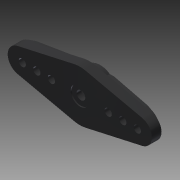
# Autodesk Inventor part: servo arm TGY-S8166M double
Saved by Autodesk Inventor 2013 (Build 170138000, 138)
## iProperties
Created: 2014-10-10
Part Number: servo arm TGY-S8166M double
Material: Acetal Resin, Black
Document SubType Name: Modeling
Designer: Masta
Density: 1.425 g/cm^3
Mass: 3.25867 g
Surface Area: 21.815 cm^2
Volume: 2.28679 cm^3
Author: Masta
Autodesk Inventor part; units mm, degrees
ref_plane "YZ Plane" through (0, 0, 0) normal (1, 0, 0) x (0, 1, 0)
ref_plane "XZ Plane" through (0, 0, 0) normal (0, 1, 0) x (-1, 0, 0)
ref_plane "XY Plane" through (0, 0, 0) normal (0, 0, 1) x (1, 0, 0)
sketch "Sketch1" plane through (0, 0, 0) normal (0, 1, 0) x (-1, 0, 0)
  line L0 (0, 0) -> (0, 8.7)
  arc A0 (0, 8.7) -> (-1.8885, 8.4926) centre (0, 0) ccw
  line L1 (0, 0) -> (-24.75, 0)
  arc A1 (-21.4226, 4.1487) -> (-24.75, 0) centre (-20.5, 0) ccw
  line L2 (-21.4226, 4.1487) -> (-1.8885, 8.4926)
  circle A2 centre (0, 0) radius 5.7
  line L3 (-23.5104, 3) -> (-4.8466, 3)
  line L4 (-3.2966, 4.65) -> (-19.1681, 4.65)
  point P0 (-9.75, 0)
  point P1 (-14.75, 0)
  point P2 (-19.75, 0)
  dimension "d0" = 8.7
  dimension "d1" = 24.75
  dimension "d2" = 4.25
  dimension "d3" = 19.75
  dimension "d4" = 5
  dimension "d5" = 5
  dimension "d6" = 11.4
  dimension "d8" = 4.65
  dimension "d9" = 3
  constraints: 10 end point, 7 point on circle, 4 point on line, 3 centre point, 2 coincident, 2 tangent, 1 line through centre, 1 parallel, 1 perpendicular, 1 vertical
  measures "d0" distance of L0.start L0.end
  measures "d1" distance of L0.start L1.end
  measures "d2" radius of A1
  measures "d3" distance of L0.start point (-19.75, 0)
  measures "d4" distance of point (-14.75, 0) point (-19.75, 0)
  measures "d5" distance of point (-9.75, 0) point (-14.75, 0)
  measures "d6" diameter of A2
  measures "d8" distance between parallel lines of L1 L4
  measures "d9" distance between parallel lines of L1 L3
extrude "Extrusion1" add sketch "Sketch1" along normal blind 3.3 contours L1 A2 L0 | A2 L4 L2 A0 L0 | L1 A1 L3 A2 | A2 L3 A1 L2 L4 picked at (-1.8582, 3.2917)
extrude "Extrusion2" add sketch "Sketch1" along normal blind 7 contours L1 A2 L0 | L0 A2 L1 | A2 L3 A1 L2 L4
hole "Hole1" at (9.75, 0, 0) at (14.75, 0, 0) at (19.75, 0, 0) direction (0, 1, 0) diameter 2.5 end through all
hole "Hole2" at (0, 0, 0) direction (0, 1, 0) diameter 3 end through all
mirror "Mirror1" about plane through (24.75, 0, 0) normal (0, 0, -1)
sketch "Sketch2" plane through (23.5104, 3.3, 3) normal (0, 0, -1) x (-1, 0, 0)
  line L0 (0, 3.7) -> (18.6638, 3.7) projected
  line L1 (0, 0) -> (0, 3.7) projected
  line L2 (0, 0) -> (18.6638, 3.7)
  point P0 (23.5104, -3.3)
  constraints: 2 end point
extrude "Extrusion3" cut sketch "Sketch2" along normal through all both and the other way through all
mirror "Mirror2" about plane through (0, 0, 0) normal (-1, 0, 0)
hole "Hole3" at (0, 7, 0) direction (0, -1, 0) diameter 7 depth 5
hole "Hole4" at (0, 0, 0) direction (0, 1, 0) diameter 6.3 depth 0.4
body "Solid1"
